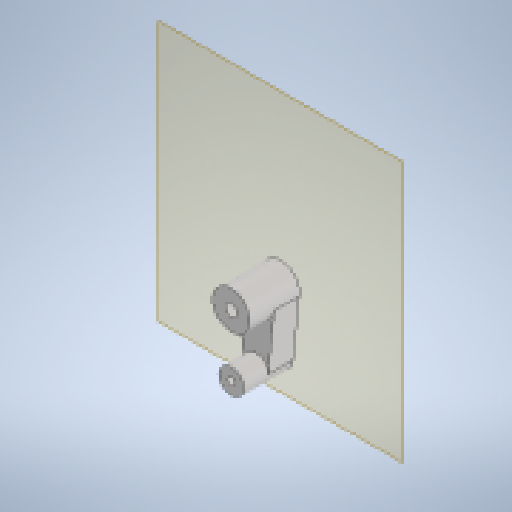
# Autodesk Inventor part: кривошип
Saved by Autodesk Inventor 2023.1 (Build 271208000, 208)
## iProperties
Created: 2024-12-17
Part Number: кривошип
Material: Типовые
Document SubType Name: Modeling
Designer: DELL
Density: 1 g/cm^3
Appearance: По умолчанию
Author: DELL
Autodesk Inventor part; units mm, degrees
ref_plane "YZ Plane" through (0, 0, 0) normal (1, 0, 0) x (0, 1, 0)
ref_plane "XZ Plane" through (0, 0, 0) normal (0, 1, 0) x (-1, 0, 0)
ref_plane "XY Plane" through (0, 0, 0) normal (0, 0, 1) x (1, 0, 0)
sketch "Эскиз1" plane through (0, 0, 0) normal (0, 0, 1) x (1, 0, 0)
  circle A0 centre (0, -14.5) radius 2.375 projected
  circle A1 centre (0, -14.5) radius 7.5
  line L0 (0, -7) -> (0, -47) construction
  arc A2 (7.5, -14.5) -> (-7.5, -14.5) centre (0, -14.5) ccw
  circle A3 centre (0, -39.5) radius 9
  spline S0 degree 1 poles (-7.5, -14.5) (-9, -39.5) knots 0 0 1 1
  spline S1 degree 1 poles (7.5, -14.5) (9, -39.5) knots 0 0 1 1
  circle A4 centre (0, -39.5) radius 1.5
  circle A5 centre (0, -39.5) radius 5
  point P0 (0, 0)
  point P1 (0, -27)
  point P2 (-7.5, -14.5)
  dimension "d1" = 15
  dimension "d3" = 18
  dimension "d4" = 3
  dimension "d9" = 10
  constraints: 5 point on circle, 4 centre point, 4 end point, 3 coincident, 1 midpoint, 1 point on line, 1 vertical, 7 other
  measures "d3" diameter of A3
  measures "d4" diameter of A4
  measures "d9" diameter of A5
extrude "Выдавливание1" add sketch "Эскиз1" along normal blind 20 contours S1 A3 S0 | A3 S1 | S0 A3
ref_plane "РабПлоскость1" through (0, 0, 0) normal (0, 0, 1) x (1, 0, 0)
sketch "Эскиз2" plane through (0, 0, 0) normal (0, 0, 1) x (1, 0, 0)
  arc A0 (-8.9721, -40.2077) -> (8.9721, -40.2077) centre (0, -39.5) ccw
  circle A1 centre (0, -39.1192) radius 1.5 construction
  line L0 (0, -39.1192) -> (0, 0.9204) construction
  line L1 (-6.4286, 47.5) -> (-19.2857, 47.5) construction
  line L2 (-19.2857, 47.5) -> (-19.2857, 42.5) construction
  line L3 (-19.2857, 42.5) -> (-24.2143, 42.5) construction
  line L4 (-24.2143, 42.5) -> (-24.2143, 36.15) construction
  line L5 (-24.2143, 36.15) -> (-22.9643, 36.15) construction
  line L6 (-22.9643, 36.15) -> (-22.9643, 33.85) construction
  line L7 (-22.9643, 33.85) -> (-24.2143, 33.85) construction
  line L8 (-24.2143, 33.85) -> (-24.2143, 27.5) construction
  line L9 (-24.2143, 27.5) -> (-27.2143, 27.5) construction
  line L10 (-27.2143, 27.5) -> (-27.2143, 33.85) construction
  line L11 (-27.2143, 33.85) -> (-28.4643, 33.85) construction
  line L12 (-28.4643, 33.85) -> (-28.4643, 36.15) construction
  line L13 (-28.4643, 36.15) -> (-27.2143, 36.15) construction
  line L14 (-27.2143, 36.15) -> (-27.2143, 42.5) construction
  line L15 (-27.2143, 42.5) -> (-32.1429, 42.5) construction
  line L16 (-32.1429, 42.5) -> (-32.1429, 47.5) construction
  line L17 (-32.1429, 47.5) -> (-45, 47.5) construction
  line L18 (-45, 47.5) -> (-45, -11.5) construction
  arc A2 (-45, -11.5) -> (-42, -14.5) centre (-42, -11.5) ccw construction
  line L19 (-42, -14.5) -> (-36.8782, -14.5) construction
  arc A3 (-33.8881, -17.2568) -> (-36.8782, -14.5) centre (-36.8782, -17.5) ccw construction
  arc A4 (-33.8881, -17.2568) -> (33.8881, -17.2568) centre (0, -14.5) ccw construction
  arc A5 (36.8782, -14.5) -> (33.8881, -17.2568) centre (36.8782, -17.5) ccw construction
  line L20 (36.8782, -14.5) -> (42, -14.5) construction
  arc A6 (42, -14.5) -> (45, -11.5) centre (42, -11.5) ccw construction
  line L21 (45, -11.5) -> (45, 47.5) construction
  line L22 (45, 47.5) -> (32.1429, 47.5) construction
  line L23 (32.1429, 47.5) -> (32.1429, 42.5) construction
  line L24 (32.1429, 42.5) -> (27.2143, 42.5) construction
  line L25 (27.2143, 42.5) -> (27.2143, 36.15) construction
  line L26 (27.2143, 36.15) -> (28.4643, 36.15) construction
  line L27 (28.4643, 36.15) -> (28.4643, 33.85) construction
  line L28 (28.4643, 33.85) -> (27.2143, 33.85) construction
  line L29 (27.2143, 33.85) -> (27.2143, 27.5) construction
  line L30 (27.2143, 27.5) -> (24.2143, 27.5) construction
  line L31 (24.2143, 27.5) -> (24.2143, 33.85) construction
  line L32 (24.2143, 33.85) -> (22.9643, 33.85) construction
  line L33 (22.9643, 33.85) -> (22.9643, 36.15) construction
  line L34 (22.9643, 36.15) -> (24.2143, 36.15) construction
  line L35 (24.2143, 36.15) -> (24.2143, 42.5) construction
  line L36 (24.2143, 42.5) -> (19.2857, 42.5) construction
  line L37 (19.2857, 42.5) -> (19.2857, 47.5) construction
  line L38 (19.2857, 47.5) -> (6.4286, 47.5) construction
  line L39 (6.4286, 47.5) -> (6.4286, 42.5) construction
  line L40 (6.4286, 42.5) -> (-6.4286, 42.5) construction
  line L41 (-6.4286, 42.5) -> (-6.4286, 47.5) construction
  circle A7 centre (0, -14.5) radius 2.375 construction
  circle A8 centre (0, -14.5) radius 5
  arc A9 (10.864, -16.2247) -> (-10.864, -16.2247) centre (0, -14.5) ccw
  line L42 (-11, -14.5) -> (-8.9721, -40.2077)
  circle A10 centre (0, -39.5) radius 9 construction
  line L43 (11, -14.5) -> (8.9721, -40.2077)
  circle A11 centre (0, -39.5) radius 1.5
  circle A12 centre (0, -6.5) radius 1.575
  circle A13 centre (8, -14.5) radius 1.575
  circle A14 centre (0, -22.5) radius 1.575
  circle A15 centre (-8, -14.5) radius 1.575
  point P0 (0, 0)
  point P1 (0, -4.925)
  point P2 (0, -3.5)
  point P3 (0, -3.5)
  point P4 (9.575, -14.5)
  point P5 (0, -24.075)
  point P6 (-9.575, -14.5)
  dimension "d22" = 3.15
  dimension "d20" = 10
  dimension "d21" = 22
  dimension "d27" = 8
  dimension "d30" = 360
  constraints: 9 point on circle, 7 coincident, 6 end point, 5 centre point, 5 point on line, 2 horizontal alignment, 2 tangent, 2 vertical alignment, 1 equal radius, 1 vertical, 23 other
  measures "d20" diameter of A8
  measures "d21" diameter of A9
  measures "d27" distance of A4.centre point (0, -6.5)
extrude "Выдавливание2" add sketch "Эскиз2" along normal blind 10 contours L42 A9 L43 A0
sketch "Эскиз3" plane through (0, 0, 0) normal (0, 0, -1) x (-1, 0, 0)
  circle A0 centre (0, -39.5) radius 4 projected
  point P0 (0, 0)
extrude "Выдавливание3" cut sketch "Эскиз3" against normal blind 10
ref_plane "РабПлоскость5" through (-8, -14.5, 0) normal (-0.7071068, 0.7071068, 0) x (0, 0, 1)
sketch "Эскиз4" plane through (-8, -14.5, 0) normal (-0.7071068, 0.7071068, 0) x (0, 0, 1)
  line L0 (10, 1.575) -> (0, 1.575) construction
  line L1 (0, 1.575) -> (0, 9.7387) construction
  line L2 (0, 9.7387) -> (10, 9.7387) construction
  line L3 (10, 9.7387) -> (10, 1.575) construction
  line L4 (10, -3.9325) -> (0, -3.9325) construction
  line L5 (0, -3.9325) -> (0, -1.575) construction
  line L6 (0, -1.575) -> (10, -1.575) construction
  line L7 (10, -1.575) -> (10, -3.9325) construction
  line L8 (0, 15.0908) -> (10, 15.0908) construction
  line L9 (10, 15.0908) -> (10, 12.8887) construction
  line L10 (10, 12.8887) -> (0, 12.8887) construction
  line L11 (0, 12.8887) -> (0, 15.0908) construction
  line L12 (10, 1.575) -> (10, -1.575) construction
  line L13 (0, 12.8887) -> (0, 9.7387) construction
  circle A0 centre (6, 5.6568) radius 1.575
  point P0 (0, 15.9099)
  dimension "d32" = 3.15
  dimension "d33" = 4
  constraints: 1 centre point
  measures "d32" diameter of A0
  measures "d33" distance from line of L3 A0.centre
extrude "Выдавливание4" cut sketch "Эскиз4" along normal blind 10
